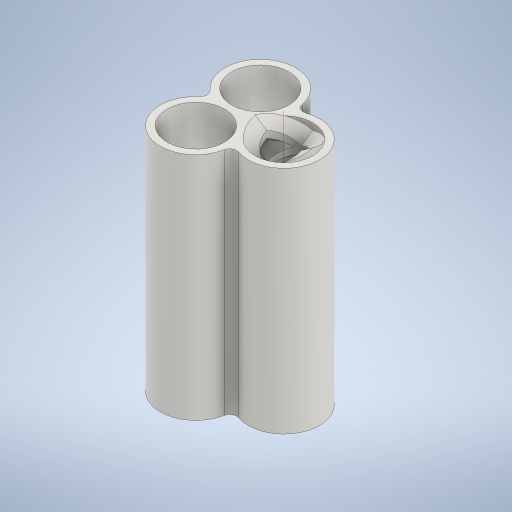
# Autodesk Inventor part: Soft Robot
Saved by Autodesk Inventor 2024.2 (Build 282272000, 272)
## iProperties
Created: 2024-02-13
Part Number: Soft Robot
Material: Generic
Document SubType Name: Modeling
Designer: jp.reyesf
Density: 1 g/cm^3
Appearance: Steel
Author: jp.reyesf
Autodesk Inventor part; units mm, degrees
ref_plane "YZ Plane" through (0, 0, 0) normal (1, 0, 0) x (0, 1, 0)
sketch "Sketch5" plane through (0, 0, 0) normal (0, 1, 0) x (-1, 0, 0)
  line L0 (0, 0) -> (-16.1658, 0) construction
  line L1 (0, 0) -> (8.0829, 14) construction
  line L2 (0, 0) -> (8.0829, -14) construction
  circle A0 centre (8.0829, 14) radius 12.5
  circle A1 centre (8.0829, 14) radius 15.5
  circle A2 centre (8.0829, -14) radius 12.5
  circle A3 centre (8.0829, -14) radius 15.5
  circle A4 centre (-16.1658, 0) radius 12.5
  circle A5 centre (-16.1658, 0) radius 15.5
  point P0 (14.735, 0)
  point P1 (-7.3675, 12.7609)
  point P2 (-7.3675, -12.7609)
  point P3 (-3.6658, 0)
  dimension "d47" = 120
  dimension "d48" = 120
  dimension "d49" = 25
  dimension "d50" = 3
  constraints: 7 coincident, 6 end point, 5 centre point, 3 equal radius, 2 equal length, 1 horizontal, 1 horizontal alignment, 1 point on line, 1 tangent, 3 other
  measures "d47" angle of L2 L0
  measures "d48" angle of L1 L0
  measures "d49" diameter of A0
  measures "d50" radial gap between concentric circles of A1 A0
extrude "Extrusion47" add sketch "Sketch5" along normal blind 100 contours A0 A5 A1 A3 | A0 A3 A1 A5 | A5 A1 | A3 A1 | A5 A3 A4 A1 | A1 A3 A5 | A1 A4 A3 A5 | A3 A5 A2 A1 | A1 A2 A5 A3 | A3 A5
fillet "Fillet7" radius 3 3 edges at (7.3675, 50, 12.7609) (-14.735, 50, 0) (7.3675, 50, -12.7609)
ref_plane "Work Plane11" through (3.6658, 0, 0) normal (0, 0, 1) x (1, 0, 0)
ref_plane "Work Plane12" through (16.1658, 0, 0) normal (0, 0, 1) x (0, 1, 0)
sketch "Sketch32" plane through (16.1658, 0, 0) normal (0, 0, 1) x (0, 1, 0)
  line L0 (100, 12.5) -> (100, -12.5) construction
  line L1 (6.501, 12.5) -> (3.501, 12.5)
  line L2 (3.501, 12.5) -> (3.501, 7.5)
  line L3 (6.501, 12.5) -> (6.501, 7.5)
  line L4 (100, 12.5) -> (100, -12.5) projected
  line L5 (6.501, 7.5) -> (3.501, 7.5)
  line L6 (100, 12.5) -> (100, -12.5) projected
  line L7 (0, 12.5) -> (0, -12.5) projected
  line L8 (3.501, 12.5) -> (0, 12.5)
  line L9 (6.501, 12.5) -> (10.0021, 12.5)
  line L10 (3.501, 7.5) -> (0, 12.5)
  line L11 (6.501, 7.5) -> (10.0021, 12.5)
  point P0 (0, 16.1658)
  point P1 (3.501, 10.5)
  point P2 (6.501, 10.5)
  dimension "d237" = 5
  dimension "d258" = 3
  dimension "d266" = 55
  constraints: 16 end point, 3 horizontal, 2 perpendicular, 2 point on line, 1 collinear, 1 parallel
  measures "d237" distance of L1.end L2.end
  measures "d258" distance of L1.start L1.end
  measures "d266" angle of L9 L11
coil "Coil4" sketch "Sketch32" operation add axis through (16.1658, 0, 0) along (0, 1, 0) pitch 23.25 turns 4 hand left
coil "Coil5" sketch "Sketch32" operation add axis through (16.1658, 0, 0) along (0, 1, 0) pitch 23.25 turns 4 hand right
ref_plane "Work Plane13" through (16.1658, 0, 0) normal (1, 0, 0) x (0, 1, 0)
mirror "Mirror3" about plane through (16.1658, 0, 0) normal (1, 0, 0) of "Coil5", "Coil4"
body "Solid22"
